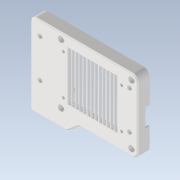
# Autodesk Inventor part: CM4_Case_Buttom
Saved by Autodesk Inventor 2022.1 (Build 261234020, 234B)
## iProperties
Created: 2022-07-26
Part Number: CM4_Case_Buttom
Material: Generisch
Document SubType Name: Modeling
Designer: Rama
Density: 1 g/cm^3
Appearance: Vorgabe
Author: Rama
Autodesk Inventor part; units mm, degrees
ref_plane "YZ Plane" through (0, 0, 0) normal (1, 0, 0) x (0, 1, 0)
ref_plane "XZ Plane" through (0, 0, 0) normal (0, 1, 0) x (-1, 0, 0)
ref_plane "XY Plane" through (0, 0, 0) normal (0, 0, 1) x (1, 0, 0)
sketch "Skizze1" plane through (0, 0, 0) normal (0, 0, 1) x (1, 0, 0)
  circle A0 centre (-59.4355, 41.65) radius 1.35 projected
  circle A1 centre (-59.433, 8.65) radius 1.35 projected
  circle A2 centre (-11.4355, 41.6536) radius 1.35 projected
  circle A3 centre (-11.433, 8.65) radius 1.35 projected
  circle A4 centre (-61.383, 0) radius 1.5 projected
  circle A5 centre (-61.383, 49) radius 1.5 projected
  circle A6 centre (-3.383, 49) radius 1.5 projected
  circle A7 centre (-3.383, 0) radius 1.5 projected
  circle A8 centre (-59.433, 8.65) radius 3.55
  circle A9 centre (-61.383, 0) radius 3.55
  circle A10 centre (-59.4355, 41.65) radius 3.55
  circle A11 centre (-61.383, 49) radius 3.55
  circle A12 centre (-3.383, 49) radius 3.55
  circle A13 centre (-11.4355, 41.6536) radius 3.55
  circle A14 centre (-11.433, 8.65) radius 3.55
  circle A15 centre (-3.383, 0) radius 3.55
  point P0 (0, 0)
  dimension "d0" = 7.1
  dimension "d1" = 7.1
  dimension "d2" = 7.1
  dimension "d3" = 7.1
  dimension "d4" = 7.1
  dimension "d5" = 7.1
  dimension "d6" = 7.1
  dimension "d7" = 7.1
  constraints: 8 centre point, 8 coincident
  measures "d0" diameter of A8
  measures "d1" diameter of A9
  measures "d2" diameter of A10
  measures "d3" diameter of A11
  measures "d4" diameter of A13
  measures "d5" diameter of A12
  measures "d6" diameter of A14
  measures "d7" diameter of A15
extrude "Extrusion1" add sketch "Skizze1" along normal blind 3.8 contours A0 | A1 | A2 | A3 | A4 | A5 | A6 | A7 | A8 | A9 | A10 | A11 | A12 | A13 | A14 | A15
sketch "Skizze2" plane through (-61.383, 0, 3.8) normal (0, 0, 1) x (1, 0, 0)
  line L0 (-20, 52.383) -> (58, 52.3726) projected
  line L1 (-20.5292, 52.3414) -> (-20, 52.383) projected
  line L2 (-21.0454, 52.2175) -> (-20.5292, 52.3414) projected
  line L3 (-21.5359, 52.0143) -> (-21.0454, 52.2175) projected
  line L4 (-21.9885, 51.7369) -> (-21.5359, 52.0143) projected
  line L5 (-22.3922, 51.3922) -> (-21.9885, 51.7369) projected
  line L6 (-22.7369, 50.9885) -> (-22.3922, 51.3922) projected
  line L7 (-23.0143, 50.5359) -> (-22.7369, 50.9885) projected
  line L8 (-23.2175, 50.0454) -> (-23.0143, 50.5359) projected
  line L9 (-23.3414, 49.5292) -> (-23.2175, 50.0454) projected
  line L10 (-23.3726, 49) -> (-23.3414, 49.5292) projected
  line L11 (-23.383, 0) -> (-23.3726, 49) projected
  line L12 (-23.3414, -0.5292) -> (-23.383, 0) projected
  line L13 (-23.2175, -1.0454) -> (-23.3414, -0.5292) projected
  line L14 (-23.0143, -1.5359) -> (-23.2175, -1.0454) projected
  line L15 (-22.7369, -1.9885) -> (-23.0143, -1.5359) projected
  line L16 (-22.3922, -2.3922) -> (-22.7369, -1.9885) projected
  line L17 (-21.9885, -2.7369) -> (-22.3922, -2.3922) projected
  line L18 (-21.5359, -3.0143) -> (-21.9885, -2.7369) projected
  line L19 (-21.0454, -3.2175) -> (-21.5359, -3.0143) projected
  line L20 (-20.5292, -3.3414) -> (-21.0454, -3.2175) projected
  line L21 (-20, -3.3726) -> (-20.5292, -3.3414) projected
  line L22 (58, -3.383) -> (-20, -3.3726) projected
  line L23 (58.5292, -3.3414) -> (58, -3.383) projected
  line L24 (59.0454, -3.2175) -> (58.5292, -3.3414) projected
  line L25 (59.5359, -3.0143) -> (59.0454, -3.2175) projected
  line L26 (59.9885, -2.7369) -> (59.5359, -3.0143) projected
  line L27 (60.3922, -2.3922) -> (59.9885, -2.7369) projected
  line L28 (60.7369, -1.9885) -> (60.3922, -2.3922) projected
  line L29 (61.0143, -1.5359) -> (60.7369, -1.9885) projected
  line L30 (61.2175, -1.0454) -> (61.0143, -1.5359) projected
  line L31 (61.3414, -0.5292) -> (61.2175, -1.0454) projected
  line L32 (61.383, 0) -> (61.3414, -0.5292) projected
  line L33 (61.383, 49) -> (61.3726, 0.0008) projected
  line L34 (61.3414, 49.5292) -> (61.383, 49) projected
  line L35 (61.2175, 50.0454) -> (61.3414, 49.5292) projected
  line L36 (61.0143, 50.5359) -> (61.2175, 50.0454) projected
  line L37 (60.7369, 50.9885) -> (61.0143, 50.5359) projected
  line L38 (60.3922, 51.3922) -> (60.7369, 50.9885) projected
  line L39 (59.9885, 51.7369) -> (60.3922, 51.3922) projected
  line L40 (59.5359, 52.0143) -> (59.9885, 51.7369) projected
  line L41 (59.0454, 52.2175) -> (59.5359, 52.0143) projected
  line L42 (58.5292, 52.3414) -> (59.0454, 52.2175) projected
  line L43 (58, 52.3726) -> (58.5292, 52.3414) projected
  line L44 (-20.3726, -3.683) -> (58.383, -3.683)
  line L45 (61.783, -0.283) -> (61.783, 49.2726)
  line L46 (58.383, 52.6726) -> (-20.3726, 52.6726)
  line L47 (-23.7726, 49.2726) -> (-23.7726, -0.283)
  arc A0 (58.383, -3.683) -> (61.783, -0.283) centre (58.383, -0.283) ccw
  arc A1 (-23.7726, -0.283) -> (-20.3726, -3.683) centre (-20.3726, -0.283) ccw
  arc A2 (-20.3726, 52.6726) -> (-23.7726, 49.2726) centre (-20.3726, 49.2726) ccw
  arc A3 (61.783, 49.2726) -> (58.383, 52.6726) centre (58.383, 49.2726) ccw
  line L48 (-20.3726, -5.283) -> (58.383, -5.283)
  line L49 (63.383, -0.283) -> (63.383, 49.2726)
  line L50 (58.383, 54.2726) -> (-20.3726, 54.2726)
  line L51 (-25.3726, 49.2726) -> (-25.3726, -0.283)
  arc A4 (-25.3726, -0.283) -> (-20.3726, -5.283) centre (-20.3726, -0.283) ccw
  arc A5 (-20.3726, 54.2726) -> (-25.3726, 49.2726) centre (-20.3726, 49.2726) ccw
  arc A6 (63.383, 49.2726) -> (58.383, 54.2726) centre (58.383, 49.2726) ccw
  arc A7 (58.383, -5.283) -> (63.383, -0.283) centre (58.383, -0.283) ccw
  dimension "d11" = 55.7557
  dimension "d12" = 84.7557
  dimension "d13" = 0.4
  dimension "d14" = 0.4
  dimension "d15" = 85.5557
  dimension "d16" = 0.3
  dimension "d17" = 0.3
  dimension "d18" = 56.3557
  dimension "d19" = 3.4
  dimension "d20" = 1.6
  dimension "d21" = 1.6
  dimension "d22" = 1.6
  dimension "d23" = 1.6
  dimension "d25" = 1.6
  constraints: 16 end point, 16 point on circle, 16 tangent, 8 centre point, 6 equal radius, 4 parallel, 2 horizontal, 2 perpendicular
  measures "d11" distance between parallel lines of L22 L0
  measures "d12" distance from line of L10.start L33
  measures "d13" distance from line of L33.start L45
  measures "d14" distance from line of L10.start L47
  measures "d15" distance between parallel lines of L45 L47
  measures "d16" distance from line of L0.end L46
  measures "d17" distance from line of L22.start L44
  measures "d18" distance between parallel lines of L46 L44
  measures "d19" radius of A0
  measures "d20" distance between parallel lines of L47 L51
  measures "d21" distance between parallel lines of L46 L50
  measures "d22" distance between parallel lines of L48 L44
  measures "d23" distance between parallel lines of L45 L49
  measures "d25" radial gap between concentric circles of A4 A1
extrude "Extrusion2" add sketch "Skizze2" against normal blind 5
sketch "Skizze3" plane through (-3.383, 0, 3.8) normal (0, 0, 1) x (1, 0, 0)
  arc A0 (0.383, -5.283) -> (5.383, -0.283) centre (0.383, -0.283) ccw projected
  line L0 (5.383, -0.283) -> (5.383, 49.2726) projected
  arc A1 (5.383, 49.2726) -> (0.383, 54.2726) centre (0.383, 49.2726) ccw projected
  line L1 (0.383, 54.2726) -> (-78.3726, 54.2726) projected
  arc A2 (-78.3726, 54.2726) -> (-83.3726, 49.2726) centre (-78.3726, 49.2726) ccw projected
  line L2 (-83.3726, 49.2726) -> (-83.3726, -0.283) projected
  arc A3 (-83.3726, -0.283) -> (-78.3726, -5.283) centre (-78.3726, -0.283) ccw projected
  line L3 (-78.3726, -5.283) -> (0.383, -5.283) projected
  arc A4 (-81.7726, -0.283) -> (-78.3726, -3.683) centre (-78.3726, -0.283) ccw projected
  line L4 (-81.7726, -0.283) -> (-81.7726, 49.2726) projected
  arc A5 (-78.3726, 52.6726) -> (-81.7726, 49.2726) centre (-78.3726, 49.2726) ccw projected
  line L5 (-78.3726, 52.6726) -> (0.383, 52.6726) projected
  arc A6 (3.783, 49.2726) -> (0.383, 52.6726) centre (0.383, 49.2726) ccw projected
  line L6 (3.783, 49.2726) -> (3.783, -0.283) projected
  arc A7 (0.383, -3.683) -> (3.783, -0.283) centre (0.383, -0.283) ccw projected
  line L7 (0.383, -3.683) -> (-78.3726, -3.683) projected
  line L8 (-52.2525, 5.75) -> (-11.8525, 5.75)
  line L9 (-11.8525, 5.75) -> (-11.8525, 46.15)
  line L10 (-11.8525, 46.15) -> (-52.2525, 46.15)
  line L11 (-52.2525, 46.15) -> (-52.2525, 5.75)
  circle A8 centre (-15.62, 25.95) radius 2.1 projected
  line L12 (-50.2525, 5.75) -> (-49.0525, 5.75)
  line L13 (-49.0525, 5.75) -> (-49.0525, 46.15)
  line L14 (-49.0525, 46.15) -> (-50.2525, 46.15)
  line L15 (-50.2525, 46.15) -> (-50.2525, 5.75)
  line L16 (-47.0525, 46.15) -> (-45.8525, 46.15)
  line L17 (-45.8525, 46.15) -> (-45.8525, 5.75)
  line L18 (-45.8525, 5.75) -> (-47.0525, 5.75)
  line L19 (-47.0525, 5.75) -> (-47.0525, 46.15)
  line L20 (-43.8525, 5.75) -> (-42.6525, 5.75)
  line L21 (-42.6525, 5.75) -> (-42.6525, 46.15)
  line L22 (-42.6525, 46.15) -> (-43.8525, 46.15)
  line L23 (-43.8525, 46.15) -> (-43.8525, 5.75)
  line L24 (-40.6525, 46.15) -> (-39.4525, 46.15)
  line L25 (-39.4525, 46.15) -> (-39.4525, 5.75)
  line L26 (-39.4525, 5.75) -> (-40.6525, 5.75)
  line L27 (-40.6525, 5.75) -> (-40.6525, 46.15)
  line L28 (-37.4525, 5.75) -> (-36.2525, 5.75)
  line L29 (-36.2525, 5.75) -> (-36.2525, 46.15)
  line L30 (-36.2525, 46.15) -> (-37.4525, 46.15)
  line L31 (-37.4525, 46.15) -> (-37.4525, 5.75)
  line L32 (-34.2525, 46.15) -> (-33.0525, 46.15)
  line L33 (-33.0525, 46.15) -> (-33.0525, 5.75)
  line L34 (-33.0525, 5.75) -> (-34.2525, 5.75)
  line L35 (-34.2525, 5.75) -> (-34.2525, 46.15)
  line L36 (-31.0525, 5.75) -> (-29.8525, 5.75)
  line L37 (-29.8525, 5.75) -> (-29.8525, 46.15)
  line L38 (-29.8525, 46.15) -> (-31.0525, 46.15)
  line L39 (-31.0525, 46.15) -> (-31.0525, 5.75)
  line L40 (-27.8525, 46.15) -> (-26.6525, 46.15)
  line L41 (-26.6525, 46.15) -> (-26.6525, 5.75)
  line L42 (-26.6525, 5.75) -> (-27.8525, 5.75)
  line L43 (-27.8525, 5.75) -> (-27.8525, 46.15)
  line L44 (-24.6525, 5.75) -> (-23.4525, 5.75)
  line L45 (-23.4525, 5.75) -> (-23.4525, 46.15)
  line L46 (-23.4525, 46.15) -> (-24.6525, 46.15)
  line L47 (-24.6525, 46.15) -> (-24.6525, 5.75)
  line L48 (-21.4525, 46.15) -> (-20.2525, 46.15)
  line L49 (-20.2525, 46.15) -> (-20.2525, 5.75)
  line L50 (-20.2525, 5.75) -> (-21.4525, 5.75)
  line L51 (-21.4525, 5.75) -> (-21.4525, 46.15)
  line L52 (-18.2525, 5.75) -> (-17.0525, 5.75)
  line L53 (-17.0525, 5.75) -> (-17.0525, 46.15)
  line L54 (-17.0525, 46.15) -> (-18.2525, 46.15)
  line L55 (-18.2525, 46.15) -> (-18.2525, 5.75)
  line L56 (-15.0525, 5.75) -> (-13.8525, 5.75)
  line L57 (-13.8525, 5.75) -> (-13.8525, 46.15)
  line L58 (-13.8525, 46.15) -> (-15.0525, 46.15)
  line L59 (-15.0525, 46.15) -> (-15.0525, 5.75)
  circle A9 centre (-56.0525, 41.65) radius 3.55 projected
  circle A10 centre (-8.0525, 41.6536) radius 3.55 projected
  point P0 (3.383, 0)
  point P1 (-52.2525, 25.95)
  point P2 (-32.0525, 5.75)
  point P3 (-11.8525, 25.95)
  point P4 (-33.6525, 46.15)
  point P5 (-30.4525, 46.15)
  point P6 (-27.2525, 46.15)
  point P7 (-24.0525, 46.15)
  point P8 (-20.8525, 46.15)
  point P9 (-17.6525, 46.15)
  point P10 (-36.8525, 46.15)
  point P11 (-40.0525, 46.15)
  point P12 (-43.2525, 46.15)
  point P13 (-46.4525, 46.15)
  point P14 (-49.6525, 46.15)
  point P15 (-14.4525, 46.15)
  dimension "d28" = 40.4
  dimension "d29" = 40.4
  dimension "d38" = 0
  dimension "d39" = 1.2
  dimension "d40" = 1.2
  dimension "d41" = 1.2
  dimension "d42" = 1.2
  dimension "d43" = 1.2
  dimension "d44" = 1.2
  dimension "d45" = 1.2
  dimension "d46" = 1.2
  dimension "d47" = 1.2
  dimension "d48" = 1.2
  dimension "d49" = 1.2
  dimension "d54" = 3.2
  dimension "d55" = 3.2
  dimension "d56" = 3.2
  dimension "d57" = 3.2
  dimension "d58" = 3.2
  dimension "d59" = 3.2
  dimension "d60" = 3.2
  dimension "d61" = 3.2
  dimension "d62" = 3.2
  dimension "d63" = 3.2
  dimension "d64" = 1.2
  dimension "d65" = 3.2
  dimension "d66" = 2
  dimension "d67" = 2
  dimension "d69" = 3.8
  dimension "d70" = 3.8
  constraints: 100 end point, 25 parallel, 14 midpoint, 12 horizontal, 12 perpendicular, 1 vertical, 31 other
  measures "d28" distance of L11.start L9.end
  measures "d29" distance of L9.end L9.start
  measures "d38" vertical distance of A8.centre point (-11.852, 25.95)
  measures "d39" distance between parallel lines of L13 L15
  measures "d40" distance between parallel lines of L17 L19
  measures "d41" distance between parallel lines of L21 L23
  measures "d42" distance between parallel lines of L25 L27
  measures "d43" distance between parallel lines of L29 L31
  measures "d44" distance between parallel lines of L33 L35
  measures "d45" distance between parallel lines of L37 L39
  measures "d46" distance between parallel lines of L41 L43
  measures "d47" distance between parallel lines of L45 L47
  measures "d48" distance between parallel lines of L49 L51
  measures "d49" distance between parallel lines of L53 L55
  measures "d54" distance of point (-33.652, 46.15) point (-30.452, 46.15)
  measures "d55" distance of point (-30.452, 46.15) point (-27.252, 46.15)
  measures "d56" distance of point (-27.252, 46.15) point (-24.052, 46.15)
  measures "d57" distance of point (-24.052, 46.15) point (-20.852, 46.15)
  measures "d58" distance of point (-20.852, 46.15) point (-17.652, 46.15)
  measures "d59" distance of point (-36.852, 46.15) point (-33.652, 46.15)
  measures "d60" distance of point (-40.052, 46.15) point (-36.852, 46.15)
  measures "d61" distance of point (-43.252, 46.15) point (-40.052, 46.15)
  measures "d62" distance of point (-46.452, 46.15) point (-43.252, 46.15)
  measures "d63" distance of point (-49.652, 46.15) point (-46.452, 46.15)
  measures "d64" distance between parallel lines of L57 L59
  measures "d65" distance of point (-17.652, 46.15) point (-14.452, 46.15)
  measures "d66" distance between parallel lines of L11 L15
  measures "d67" distance between parallel lines of L57 L9
  measures "d69" distance from line of A10.centre L9
  measures "d70" distance from line of A9.centre L11
extrude "Extrusion3" add sketch "Skizze3" along normal blind 2.6 contours L3 A3 L2 A2 L1 A1 L0 A0 | L4 A5 L5 A6 L6 A7 L7 A4 | A9 | A10
sketch "Skizze4" plane through (-3.383, 0, 6.4) normal (0, 0, 1) x (1, 0, 0)
  line L0 (-49.0525, 5.75) -> (-49.0525, 46.15) projected
  line L1 (-50.2525, 46.15) -> (-50.2525, 5.75) projected
  line L2 (5.383, -0.283) -> (5.383, 49.2726) projected
  arc A0 (5.383, 49.2726) -> (0.383, 54.2726) centre (0.383, 49.2726) ccw projected
  line L3 (0.383, 54.2726) -> (-78.3726, 54.2726) projected
  arc A1 (-78.3726, 54.2726) -> (-83.3726, 49.2726) centre (-78.3726, 49.2726) ccw projected
  line L4 (-83.3726, 49.2726) -> (-83.3726, -0.283) projected
  arc A2 (-83.3726, -0.283) -> (-78.3726, -5.283) centre (-78.3726, -0.283) ccw projected
  line L5 (-78.3726, -5.283) -> (0.383, -5.283) projected
  arc A3 (0.383, -5.283) -> (5.383, -0.283) centre (0.383, -0.283) ccw projected
  line L6 (-11.8525, 46.15) -> (-11.8525, 5.75) projected
  line L7 (-11.8525, 5.75) -> (-52.2525, 5.75) projected
  line L8 (-52.2525, 5.75) -> (-52.2525, 46.15) projected
  line L9 (-52.2525, 46.15) -> (-11.8525, 46.15) projected
  line L10 (-47.0525, 5.75) -> (-47.0525, 46.15) projected
  line L11 (-45.8525, 46.15) -> (-45.8525, 5.75) projected
  line L12 (-43.8525, 46.15) -> (-43.8525, 5.75) projected
  line L13 (-42.6525, 5.75) -> (-42.6525, 46.15) projected
  line L14 (-40.6525, 5.75) -> (-40.6525, 46.15) projected
  line L15 (-39.4525, 46.15) -> (-39.4525, 5.75) projected
  line L16 (-37.4525, 46.15) -> (-37.4525, 5.75) projected
  line L17 (-36.2525, 5.75) -> (-36.2525, 46.15) projected
  line L18 (-34.2525, 5.75) -> (-34.2525, 46.15) projected
  line L19 (-33.0525, 46.15) -> (-33.0525, 5.75) projected
  line L20 (-31.0525, 46.15) -> (-31.0525, 5.75) projected
  line L21 (-29.8525, 5.75) -> (-29.8525, 46.15) projected
  line L22 (-27.8525, 5.75) -> (-27.8525, 46.15) projected
  line L23 (-26.6525, 46.15) -> (-26.6525, 5.75) projected
  line L24 (-24.6525, 46.15) -> (-24.6525, 5.75) projected
  line L25 (-23.4525, 5.75) -> (-23.4525, 46.15) projected
  line L26 (-21.4525, 5.75) -> (-21.4525, 46.15) projected
  line L27 (-20.2525, 46.15) -> (-20.2525, 5.75) projected
  line L28 (-18.2525, 46.15) -> (-18.2525, 5.75) projected
  line L29 (-17.0525, 5.75) -> (-17.0525, 46.15) projected
  line L30 (-15.0525, 46.15) -> (-15.0525, 5.75) projected
  line L31 (-13.8525, 5.75) -> (-13.8525, 46.15) projected
  point P0 (3.383, 0)
  point P1 (-49.0525, 5.75)
  point P2 (-50.2525, 5.75)
  constraints: 2 other
extrude "Extrusion4" add sketch "Skizze4" along normal blind 2.2 contours L7 L1 L9 L0 | L10 L9 L11 L7 | L12 L9 L13 L7 | L14 L9 L15 L7 | L16 L9 L17 L7 | L18 L9 L19 L7 | L20 L9 L21 L7 | L22 L9 L23 L7 | L24 L9 L25 L7 | L26 L9 L27 L7 | L28 L9 L29 L7 | L30 L9 L31 L7 | A3 L5 A2 L4 A1 L3 A0 L2
sketch "Skizze5" plane through (-3.383, 0, 8.6) normal (0, 0, 1) x (1, 0, 0)
  circle A0 centre (0, 0) radius 3.55 projected
  circle A1 centre (-58, 0) radius 3.55 projected
  circle A2 centre (-56.05, 8.65) radius 3.55 projected
  circle A3 centre (0, 49) radius 3.55 projected
  circle A4 centre (-8.0525, 41.6536) radius 3.55 projected
  circle A5 centre (-56.0525, 41.65) radius 3.55 projected
  circle A6 centre (-58, 49) radius 3.55 projected
  circle A7 centre (-8.05, 8.65) radius 3.55 projected
  point P0 (3.383, 0)
hole "Bohrung1" at (-61.383, 0, 8.6) at (-3.383, 0, 8.6) at (-3.383, 49, 8.6) at (-61.383, 49, 8.6) direction (0, 0, -1) diameter 3.3 end through all counterbore diameter 4.7 counterbore depth 5
hole "Bohrung2" at (-59.4355, 41.65, 8.6) at (-59.433, 8.65, 8.6) at (-11.433, 8.65, 8.6) at (-11.4355, 41.6536, 8.6) direction (0, 0, -1) diameter 2.5 end through all
sketch "Skizze6" plane through (-3.383, 0, 3.8) normal (0, 0, -1) x (-1, 0, 0)
  line L0 (75.3726, 42.6448) -> (1.617, 42.6448)
  line L1 (1.617, 42.6448) -> (1.617, 11.1448)
  line L2 (1.617, 11.1448) -> (75.3726, 11.1448)
  line L3 (75.3726, 11.1448) -> (75.3726, 42.6448)
  line L4 (-5.383, 49.2726) -> (-5.383, -0.283) projected
  line L5 (83.3726, -0.283) -> (83.3726, 49.2726) projected
  point P0 (-3.383, 0)
  point P1 (-5.383, 24.4948)
  point P2 (1.617, 26.8948)
  point P3 (-5.383, 24.4948)
  dimension "d89" = 31.5
  dimension "d91" = 7
  dimension "d92" = 8
  dimension "d93" = 2.4
  constraints: 8 end point, 3 midpoint, 2 parallel, 1 horizontal, 1 perpendicular
  measures "d89" distance of L1.end L0.end
  measures "d91" distance between parallel lines of L4 L1
  measures "d92" distance between parallel lines of L5 L3
  measures "d93" vertical distance of point (1.617, 26.895) point (-5.383, 24.495)
hole "Bohrung3" at (-5, 42.6448, 3.8) at (-5, 11.1448, 3.8) at (-78.7557, 11.1448, 3.8) at (-78.7557, 42.6448, 3.8) direction (0, 0, 1) diameter 3.3 end through all counterbore diameter 5.8 counterbore depth 3.2
chamfer "Fase1" distance 0.4 angle 45 36 edges at (-62.983, 8.65, 0) (-64.933, 0, 0) (-62.9855, 41.65, 0) (-64.933, 49, 0) (-14.9855, 41.6536, 0) (-6.933, 49, 0) (-14.983, 8.65, 0) (-6.933, 0, 0) (-18.4355, 25.95, 6.4) (-17.2355, 25.95, 6.4) (-21.6355, 25.95, 6.4) (-20.4355, 25.95, 6.4) (-15.2355, 25.95, 3.8) (-35.4355, 46.15, 3.8) (-35.4355, 5.75, 3.8) (-55.6355, 25.95, 3.8) (-23.6355, 25.95, 6.4) (-24.8355, 25.95, 6.4) (-28.0355, 25.95, 6.4) (-26.8355, 25.95, 6.4) (-31.2355, 25.95, 6.4) (-30.0355, 25.95, 6.4) (-34.4355, 25.95, 6.4) (-33.2355, 25.95, 6.4) (-37.6355, 25.95, 6.4) (-36.4355, 25.95, 6.4) (-40.8355, 25.95, 6.4) (-39.6355, 25.95, 6.4) (-44.0355, 25.95, 6.4) (-42.8355, 25.95, 6.4) (-47.2355, 25.95, 6.4) (-46.0355, 25.95, 6.4) (-50.4355, 25.95, 6.4) (-49.2355, 25.95, 6.4) (-52.4355, 25.95, 6.4) (-53.6355, 25.95, 6.4)
chamfer "Fase2" distance 0.4 angle 45 52 edges at (-53.6355, 25.95, 8.6) (-52.4355, 25.95, 8.6) (-50.4355, 25.95, 8.6) (-49.2355, 25.95, 8.6) (-47.2355, 25.95, 8.6) (-46.0355, 25.95, 8.6) (-44.0355, 25.95, 8.6) (-42.8355, 25.95, 8.6) (-40.8355, 25.95, 8.6) (-39.6355, 25.95, 8.6) (-37.6355, 25.95, 8.6) (-36.4355, 25.95, 8.6) (-34.4355, 25.95, 8.6) (-33.2355, 25.95, 8.6) (-31.2355, 25.95, 8.6) (-30.0355, 25.95, 8.6) (-28.0355, 25.95, 8.6) (-26.8355, 25.95, 8.6) (-24.8355, 25.95, 8.6) (-23.6355, 25.95, 8.6) (-21.6355, 25.95, 8.6) (-20.4355, 25.95, 8.6) (-18.4355, 25.95, 8.6) (-17.2355, 25.95, 8.6) (-15.2355, 25.95, 8.6) (-55.6355, 25.95, 8.6) (-54.6355, 5.75, 8.6) (-51.4355, 5.75, 8.6) (-48.2355, 5.75, 8.6) (-45.0355, 5.75, 8.6) (-41.8355, 5.75, 8.6) (-38.6355, 5.75, 8.6) (-35.4355, 5.75, 8.6) (-32.2355, 5.75, 8.6) (-29.0355, 5.75, 8.6) (-25.8355, 5.75, 8.6) (-22.6355, 5.75, 8.6) (-19.4355, 5.75, 8.6) (-16.2355, 5.75, 8.6) (-16.2355, 46.15, 8.6) (-19.4355, 46.15, 8.6) (-22.6355, 46.15, 8.6) (-25.8355, 46.15, 8.6) (-29.0355, 46.15, 8.6) (-32.2355, 46.15, 8.6) (-35.4355, 46.15, 8.6) (-38.6355, 46.15, 8.6) (-41.8355, 46.15, 8.6) (-45.0355, 46.15, 8.6) (-48.2355, 46.15, 8.6) (-51.4355, 46.15, 8.6) (-54.6355, 46.15, 8.6)
sketch "Skizze7" plane through (-61.383, 0, -1.2) normal (0, 0, -1) x (-1, 0, 0)
  arc A0 (-63.383, -0.283) -> (-58.383, -5.283) centre (-58.383, -0.283) ccw projected
  line L0 (-58.383, -5.283) -> (20.3726, -5.283) projected
  arc A1 (20.3726, -5.283) -> (25.3726, -0.283) centre (20.3726, -0.283) ccw projected
  line L1 (25.3726, -0.283) -> (25.3726, 49.2726) projected
  arc A2 (25.3726, 49.2726) -> (20.3726, 54.2726) centre (20.3726, 49.2726) ccw projected
  line L2 (20.3726, 54.2726) -> (-58.383, 54.2726) projected
  arc A3 (-58.383, 54.2726) -> (-63.383, 49.2726) centre (-58.383, 49.2726) ccw projected
  line L3 (-63.383, 49.2726) -> (-63.383, -0.283) projected
  arc A4 (20.3726, -3.683) -> (23.7726, -0.283) centre (20.3726, -0.283) ccw projected
  line L4 (20.3726, -3.683) -> (-58.383, -3.683) projected
  arc A5 (-61.783, -0.283) -> (-58.383, -3.683) centre (-58.383, -0.283) ccw projected
  line L5 (-61.783, -0.283) -> (-61.783, 49.2726) projected
  arc A6 (-58.383, 52.6726) -> (-61.783, 49.2726) centre (-58.383, 49.2726) ccw projected
  line L6 (-58.383, 52.6726) -> (20.3726, 52.6726) projected
  arc A7 (23.7726, 49.2726) -> (20.3726, 52.6726) centre (20.3726, 49.2726) ccw projected
  line L7 (23.7726, 49.2726) -> (23.7726, -0.283) projected
  line L8 (25.3726, 49.2726) -> (25.3726, -0.283) projected
  line L9 (25.3726, 6.4318) -> (-5.8274, 6.4318)
  line L10 (-5.8274, 6.4318) -> (-5.8274, -13.283)
  line L11 (-5.8274, -13.283) -> (25.3726, -13.283)
  line L12 (25.3726, -13.283) -> (25.3726, 6.4318)
  line L13 (23.7726, 49.2726) -> (23.7726, -0.283) projected
  line L14 (23.7726, 8.4987) -> (-4.2274, 8.4987)
  line L15 (-4.2274, 8.4987) -> (-4.2274, -11.683)
  line L16 (-4.2274, -11.683) -> (23.7726, -11.683)
  line L17 (23.7726, -11.683) -> (23.7726, 8.4987)
  line L18 (23.7726, -9.883) -> (-4.2274, -9.883)
  point P0 (-61.383, 0)
  point P1 (-5.8274, -5.283)
  point P2 (25.3726, -0.283)
  dimension "d107" = 8
  dimension "d108" = 29.6
  dimension "d109" = 1.6
  dimension "d110" = 1.6
  dimension "d111" = 1.8
  dimension "d114" = 1.6
  constraints: 18 end point, 4 parallel, 4 point on line, 3 perpendicular, 2 horizontal
  measures "d107" distance between parallel lines of L0 L11
  measures "d108" distance between parallel lines of L7 L10
  measures "d109" distance between parallel lines of L10 L15
  measures "d110" distance between parallel lines of L11 L16
  measures "d111" distance between parallel lines of L16 L18
  measures "d114" distance between parallel lines of L4 L0
extrude "Extrusion5" add sketch "Skizze7" against normal blind 3.2 contours L0 L15 L16 L17 A1 L12 L11 L10 | L0 A1 L17 L18 L15
sketch "Skizze8" plane through (-61.383, 0, -1.2) normal (0, 0, -1) x (-1, 0, 0)
  line L0 (23.7726, -9.883) -> (-4.2274, -9.883) projected
  line L1 (6.3726, -9.883) -> (0.5726, -9.883)
  line L2 (0.5726, -9.883) -> (0.5726, -7.283)
  line L3 (0.5726, -7.283) -> (6.3726, -7.283)
  line L4 (6.3726, -7.283) -> (6.3726, -9.883)
  line L5 (23.7726, -9.883) -> (23.7726, -11.683) projected
  line L6 (-4.2274, -11.683) -> (-4.2274, -9.883) projected
  line L7 (23.7726, -11.683) -> (-4.2274, -11.683) projected
  point P0 (-61.383, 0)
  point P1 (0.5726, -9.883)
  dimension "d115" = 17.4
  dimension "d116" = 4.8
  dimension "d117" = 4.4
  constraints: 8 end point, 2 parallel, 1 horizontal, 1 perpendicular, 1 point on line
  measures "d115" distance between parallel lines of L5 L4
  measures "d116" distance between parallel lines of L6 L2
  measures "d117" distance between parallel lines of L7 L3
extrude "Extrusion6" cut sketch "Skizze8" against normal through all contours L0 L2 L3 L4
sketch "Skizze9" plane through (-61.383, 0, 2) normal (0, 0, 1) x (1, 0, 0)
  line L0 (-6.3726, -9.883) -> (-6.3726, -7.283) projected
  line L1 (-6.3726, -7.283) -> (-0.5726, -7.283) projected
  line L2 (-0.5726, -7.283) -> (-0.5726, -9.883) projected
  line L3 (-0.5726, -9.883) -> (4.2274, -9.883) projected
  line L4 (4.2274, -9.883) -> (4.2274, -11.683) projected
  line L5 (4.2274, -11.683) -> (-23.7726, -11.683) projected
  line L6 (-23.7726, -11.683) -> (-23.7726, -9.883) projected
  line L7 (-23.7726, -9.883) -> (-6.3726, -9.883) projected
  line L8 (5.8274, -13.283) -> (5.8274, -5.283) projected
  line L9 (-20.3726, -5.283) -> (5.8274, -5.283) projected
  arc A0 (-25.3726, -0.283) -> (-20.3726, -5.283) centre (-20.3726, -0.283) ccw projected
  line L10 (-25.3726, -0.283) -> (-25.3726, -13.283) projected
  line L11 (-25.3726, -13.283) -> (5.8274, -13.283) projected
  point P0 (61.383, 0)
extrude "Extrusion7" add sketch "Skizze9" along normal up to surface (6.6 mm away) contours L0 L1 L2 L3 L4 L5 L6 L7 | L11 L10 A0 L9 L8
fillet "Rundung1" radius 3 1 edges at (-55.5557, -5.283, 3.7)
fillet "Rundung2" radius 1.6 2 edges at (-55.5557, -13.283, 3.7) (-86.7557, -13.283, 3.7)
sketch "Skizze10" plane through (-3.383, 0, 8.6) normal (0, 0, 1) x (1, 0, 0)
  arc A0 (-83.3726, -11.683) -> (-81.7726, -13.283) centre (-81.7726, -11.683) ccw projected
  line L0 (-53.7726, -13.283) -> (-81.7726, -13.283) projected
  arc A1 (-53.7726, -13.283) -> (-52.1726, -11.683) centre (-53.7726, -11.683) ccw projected
  line L1 (-52.1726, -8.283) -> (-52.1726, -11.683) projected
  arc A2 (-49.1726, -5.283) -> (-52.1726, -8.283) centre (-49.1726, -8.283) ccw projected
  line L2 (-49.1726, -5.283) -> (0.383, -5.283) projected
  arc A3 (0.383, -5.283) -> (5.383, -0.283) centre (0.383, -0.283) ccw projected
  line L3 (5.383, -0.283) -> (5.383, 49.2726) projected
  arc A4 (5.383, 49.2726) -> (0.383, 54.2726) centre (0.383, 49.2726) ccw projected
  line L4 (0.383, 54.2726) -> (-78.3726, 54.2726) projected
  arc A5 (-78.3726, 54.2726) -> (-83.3726, 49.2726) centre (-78.3726, 49.2726) ccw projected
  line L5 (-83.3726, 49.2726) -> (-83.3726, -11.683) projected
  line L6 (-11.4525, 5.35) -> (-11.4525, 46.55) projected
  line L7 (-14.2525, 5.35) -> (-11.4525, 5.35) projected
  line L8 (-14.2525, 46.55) -> (-14.2525, 5.35) projected
  line L9 (-11.4525, 46.55) -> (-14.2525, 46.55) projected
  line L10 (-17.8525, 5.35) -> (-17.8525, 46.55) projected
  line L11 (-20.6525, 5.35) -> (-17.8525, 5.35) projected
  line L12 (-20.6525, 46.55) -> (-20.6525, 5.35) projected
  line L13 (-17.8525, 46.55) -> (-20.6525, 46.55) projected
  line L14 (-24.2525, 5.35) -> (-24.2525, 46.55) projected
  line L15 (-27.0525, 5.35) -> (-24.2525, 5.35) projected
  line L16 (-27.0525, 46.55) -> (-27.0525, 5.35) projected
  line L17 (-24.2525, 46.55) -> (-27.0525, 46.55) projected
  line L18 (-30.6525, 5.35) -> (-30.6525, 46.55) projected
  line L19 (-33.4525, 5.35) -> (-30.6525, 5.35) projected
  line L20 (-33.4525, 46.55) -> (-33.4525, 5.35) projected
  line L21 (-30.6525, 46.55) -> (-33.4525, 46.55) projected
  line L22 (-37.0525, 5.35) -> (-37.0525, 46.55) projected
  line L23 (-39.8525, 5.35) -> (-37.0525, 5.35) projected
  line L24 (-39.8525, 46.55) -> (-39.8525, 5.35) projected
  line L25 (-37.0525, 46.55) -> (-39.8525, 46.55) projected
  line L26 (-43.4525, 5.35) -> (-43.4525, 46.55) projected
  line L27 (-46.2525, 5.35) -> (-43.4525, 5.35) projected
  line L28 (-46.2525, 46.55) -> (-46.2525, 5.35) projected
  line L29 (-43.4525, 46.55) -> (-46.2525, 46.55) projected
  line L30 (-52.6525, 46.55) -> (-52.6525, 5.35) projected
  line L31 (-49.8525, 46.55) -> (-52.6525, 46.55) projected
  line L32 (-49.8525, 5.35) -> (-49.8525, 46.55) projected
  line L33 (-52.6525, 5.35) -> (-49.8525, 5.35) projected
  circle A6 centre (-75.3726, 11.1448) radius 1.65 projected
  circle A7 centre (-1.617, 42.6448) radius 1.65 projected
  circle A8 centre (-1.617, 11.1448) radius 1.65 projected
  circle A9 centre (-75.3726, 42.6448) radius 1.65 projected
  circle A10 centre (-8.05, 8.65) radius 1.25 projected
  circle A11 centre (-56.0525, 41.65) radius 1.25 projected
  circle A12 centre (-56.05, 8.65) radius 1.25 projected
  circle A13 centre (-8.0525, 41.6536) radius 1.25 projected
  circle A14 centre (0, 49) radius 2.35 projected
  circle A15 centre (-58, 0) radius 2.35 projected
  circle A16 centre (0, 0) radius 2.35 projected
  circle A17 centre (-58, 49) radius 2.35 projected
  line L34 (-46.6525, 5.35) -> (-46.6525, 46.55) projected
  line L35 (-49.4525, 5.35) -> (-46.6525, 5.35) projected
  line L36 (-49.4525, 46.55) -> (-49.4525, 5.35) projected
  line L37 (-46.6525, 46.55) -> (-49.4525, 46.55) projected
  line L38 (-40.2525, 5.35) -> (-40.2525, 46.55) projected
  line L39 (-43.0525, 5.35) -> (-40.2525, 5.35) projected
  line L40 (-43.0525, 46.55) -> (-43.0525, 5.35) projected
  line L41 (-40.2525, 46.55) -> (-43.0525, 46.55) projected
  line L42 (-33.8525, 5.35) -> (-33.8525, 46.55) projected
  line L43 (-36.6525, 5.35) -> (-33.8525, 5.35) projected
  line L44 (-36.6525, 46.55) -> (-36.6525, 5.35) projected
  line L45 (-33.8525, 46.55) -> (-36.6525, 46.55) projected
  line L46 (-27.4525, 5.35) -> (-27.4525, 46.55) projected
  line L47 (-30.2525, 5.35) -> (-27.4525, 5.35) projected
  line L48 (-30.2525, 46.55) -> (-30.2525, 5.35) projected
  line L49 (-27.4525, 46.55) -> (-30.2525, 46.55) projected
  line L50 (-21.0525, 5.35) -> (-21.0525, 46.55) projected
  line L51 (-23.8525, 5.35) -> (-21.0525, 5.35) projected
  line L52 (-23.8525, 46.55) -> (-23.8525, 5.35) projected
  line L53 (-21.0525, 46.55) -> (-23.8525, 46.55) projected
  line L54 (-14.6525, 5.35) -> (-14.6525, 46.55) projected
  line L55 (-17.4525, 5.35) -> (-14.6525, 5.35) projected
  line L56 (-17.4525, 46.55) -> (-17.4525, 5.35) projected
  line L57 (-14.6525, 46.55) -> (-17.4525, 46.55) projected
  line L58 (0.9112, 45.9847) -> (5.383, 45.9847) projected
  line L59 (5.383, 49.2726) -> (5.383, 45.9847) projected
  arc A18 (5.383, 49.2726) -> (0.383, 54.2726) centre (0.383, 49.2726) ccw projected
  line L60 (-3.0834, 54.2726) -> (0.383, 54.2726) projected
  line L61 (-3.0834, 54.2726) -> (-3.0834, 49.6442) projected
  arc A19 (0.9112, 45.9847) -> (-3.0834, 49.6442) centre (0, 49) ccw projected
  line L62 (-41.7726, -3.683) -> (-3.15, -3.683) projected
  arc A20 (-41.7726, -3.683) -> (-44.6679, -4.7085) centre (-41.7726, -8.283) ccw projected
  line L63 (-53.3873, -11.771) -> (-44.6679, -4.7085) projected
  arc A21 (-54.2685, -12.083) -> (-53.3873, -11.771) centre (-54.2685, -10.683) ccw projected
  line L64 (-81.7726, -12.083) -> (-54.2685, -12.083) projected
  line L65 (-81.7726, -9.883) -> (-81.7726, -12.083) projected
  line L66 (-81.7726, -9.883) -> (-83.3726, -9.883) projected
  line L67 (-83.3726, -12.083) -> (-83.3726, -9.883) projected
  arc A22 (-83.3726, -12.083) -> (-81.7726, -13.683) centre (-81.7726, -12.083) ccw projected
  line L68 (-54.2685, -13.683) -> (-81.7726, -13.683) projected
  arc A23 (-54.2685, -13.683) -> (-52.3803, -13.0143) centre (-54.2685, -10.683) ccw projected
  line L69 (-43.6608, -5.9518) -> (-52.3803, -13.0143) projected
  arc A24 (-41.7726, -5.283) -> (-43.6608, -5.9518) centre (-41.7726, -8.283) ccw projected
  line L70 (0.383, -5.283) -> (-41.7726, -5.283) projected
  arc A25 (0.383, -5.283) -> (5.383, -0.283) centre (0.383, -0.283) ccw projected
  line L71 (5.383, 36.6777) -> (5.383, -0.283) projected
  line L72 (3.783, 36.6777) -> (5.383, 36.6777) projected
  line L73 (3.783, 3.15) -> (3.783, 36.6777) projected
  line L74 (3.783, 3.15) -> (0, 3.15) projected
  arc A26 (-3.15, 0) -> (0, 3.15) centre (0, 0) ccw projected
  line L75 (-3.15, 0) -> (-3.15, -3.683) projected
  point P0 (3.383, 0)
  point P1 (-45.3772, -5.283)
  point P2 (-52.1726, -10.7871)
extrude "Extrusion8" add sketch "Skizze10" against normal up to surface (9.8 mm away) contours A0 L0 A1 L1 L63 L2 A24 L69 A23 L68 A22 L67
sketch "Skizze12" plane through (-3.383, 0, 3.8) normal (0, 0, -1) x (-1, 0, 0)
  arc A0 (52.1726, -8.283) -> (49.1726, -5.283) centre (49.1726, -8.283) ccw projected
  line L0 (49.1726, -5.283) -> (-0.383, -5.283) projected
  line L1 (53.2788, -11.683) -> (53.3873, -11.771) projected
  line L2 (52.1726, -8.283) -> (52.1726, -10.7871) projected
  arc A1 (52.1726, -8.283) -> (49.1726, -5.283) centre (49.1726, -8.283) ccw projected
  line L3 (45.3772, -5.283) -> (49.1726, -5.283) projected
  line L4 (44.6679, -4.7085) -> (52.9726, -11.4351) projected
  point P0 (-3.383, 0)
  point P1 (52.1726, -3.683)
  point P2 (52.1726, -11.683)
extrude "Extrusion10" add sketch "Skizze12" against normal up to surface (4.8 mm away)
move faces "Verschieben1" translate (0, 0, 1) faces at (-70.0223, -11.083, 2)
chamfer "Fase4" distance 1 angle 45 7 edges at (-42.3778, 54.2726, 8.6) (-85.2912, 52.8082, 8.6) (-86.7557, 18.5948, 8.6) (-24.0778, -5.283, 8.6) (0.5355, -3.8186, 8.6) (2, 24.4948, 8.6) (0.5355, 52.8082, 8.6)
chamfer "Fase5" distance 0.6 angle 45 4 edges at (-59.4355, 42.9, 0) (-59.433, 9.9, 0) (-11.433, 9.9, 0) (-11.4355, 42.9036, 0)
sketch "Skizze13" plane through (-61.383, 0, -1.2) normal (0, 0, -1) x (-1, 0, 0)
  line L0 (-60.7952, 14.6356) -> (-48.019, 14.6356) projected
  line L1 (-60.7952, 21.8746) -> (-60.7952, 14.6356) projected
  line L2 (-61.8366, 22.916) -> (-60.7952, 21.8746) projected
  line L3 (-61.8366, 29.0882) -> (-61.8366, 22.916) projected
  line L4 (-48.019, 29.0882) -> (-61.8366, 29.0882) projected
  line L5 (-48.019, 14.6356) -> (-48.019, 29.0882) projected
  line L6 (-5.8274, -8.283) -> (-5.8274, -10.7871) projected
  line L7 (20.3726, -3.683) -> (-58.383, -3.683) projected
  arc A0 (-61.783, -0.283) -> (-58.383, -3.683) centre (-58.383, -0.283) ccw projected
  line L8 (-61.783, -0.283) -> (-61.783, 49.2726) projected
  arc A1 (-58.383, 52.6726) -> (-61.783, 49.2726) centre (-58.383, 49.2726) ccw projected
  line L9 (-58.383, 52.6726) -> (20.3726, 52.6726) projected
  arc A2 (23.7726, 49.2726) -> (20.3726, 52.6726) centre (20.3726, 49.2726) ccw projected
  line L10 (23.7726, 49.2726) -> (23.7726, -0.283) projected
  arc A3 (20.3726, -3.683) -> (23.7726, -0.283) centre (20.3726, -0.283) ccw projected
  line L11 (0.5726, -9.883) -> (0.5726, -7.283) projected
  line L12 (0.5726, -7.283) -> (6.3726, -7.283) projected
  line L13 (6.3726, -7.283) -> (6.3726, -9.883) projected
  line L14 (6.3726, -9.883) -> (23.7726, -9.883) projected
  line L15 (23.7726, -9.883) -> (23.7726, -11.683) projected
  line L16 (23.7726, -11.683) -> (-4.2274, -11.683) projected
  line L17 (-4.2274, -11.683) -> (-4.2274, -9.883) projected
  line L18 (-4.2274, -9.883) -> (0.5726, -9.883) projected
  line L19 (25.3726, -12.083) -> (25.3726, 49.2726) projected
  arc A4 (25.3726, 49.2726) -> (20.3726, 54.2726) centre (20.3726, 49.2726) ccw projected
  line L20 (20.3726, 54.2726) -> (-58.383, 54.2726) projected
  arc A5 (-58.383, 54.2726) -> (-63.383, 49.2726) centre (-58.383, 49.2726) ccw projected
  line L21 (-63.383, 49.2726) -> (-63.383, -0.283) projected
  arc A6 (-63.383, -0.283) -> (-58.383, -5.283) centre (-58.383, -0.283) ccw projected
  line L22 (-58.383, -5.283) -> (-16.2274, -5.283) projected
  line L23 (-51.8157, 29.3882) -> (-69.5161, 29.3882)
  line L24 (-69.5161, 29.3882) -> (-69.5161, 14.3356)
  line L25 (-69.5161, 14.3356) -> (-51.8157, 14.3356)
  line L26 (-51.8157, 14.3356) -> (-51.8157, 29.3882)
  line L27 (-12.6228, -5.283) -> (-8.8274, -5.283) projected
  arc A7 (-5.8274, -8.283) -> (-8.8274, -5.283) centre (-8.8274, -8.283) ccw projected
  line L28 (-5.8274, -10.7871) -> (-12.6228, -5.283) projected
  arc A8 (-14.3392, -5.9518) -> (-16.2274, -5.283) centre (-16.2274, -8.283) ccw projected
  line L29 (-14.3392, -5.9518) -> (-5.6198, -13.0143) projected
  arc A9 (-5.6198, -13.0143) -> (-3.7315, -13.683) centre (-3.7315, -10.683) ccw projected
  line L30 (-3.7315, -13.683) -> (23.7726, -13.683) projected
  arc A10 (23.7726, -13.683) -> (25.3726, -12.083) centre (23.7726, -12.083) ccw projected
  point P0 (-61.383, 0)
  point P1 (-61.783, 29.0882)
  point P2 (-61.783, 29.3882)
  point P3 (-63.383, 29.3882)
  point P4 (-63.383, 14.3356)
  point P5 (-61.783, 14.3356)
  point P6 (-61.783, 22.8624)
  dimension "d143" = 0.3
  dimension "d144" = 0.3
  constraints: 8 end point, 2 parallel, 1 horizontal, 1 perpendicular
  measures "d143" distance between parallel lines of L4 L23
  measures "d144" distance between parallel lines of L25 L0
extrude "Extrusion11" cut sketch "Skizze13" against normal blind 2.6 contours L8 L25 L21 L23 L4 L3 L2 | L2 L3 L4 L8
chamfer "Fase6" distance 1.2 angle 45 1 edges at (2, 21.8619, 1.4)
sketch "Skizze14" plane through (-61.383, 0, -1.2) normal (0, 0, -1) x (-1, 0, 0)
  line L0 (-61.783, 14.3356) -> (-63.383, 14.3356) projected
  line L1 (-63.383, 14.3356) -> (-63.383, -0.283) projected
  arc A0 (-63.383, -0.283) -> (-58.383, -5.283) centre (-58.383, -0.283) ccw projected
  line L2 (-58.383, -5.283) -> (-16.2274, -5.283) projected
  arc A1 (-14.3392, -5.9518) -> (-16.2274, -5.283) centre (-16.2274, -8.283) ccw projected
  line L3 (-14.3392, -5.9518) -> (-5.6198, -13.0143) projected
  arc A2 (-5.6198, -13.0143) -> (-3.7315, -13.683) centre (-3.7315, -10.683) ccw projected
  line L4 (-3.7315, -13.683) -> (23.7726, -13.683) projected
  arc A3 (23.7726, -13.683) -> (25.3726, -12.083) centre (23.7726, -12.083) ccw projected
  line L5 (25.3726, -12.083) -> (25.3726, 49.2726) projected
  arc A4 (25.3726, 49.2726) -> (20.3726, 54.2726) centre (20.3726, 49.2726) ccw projected
  line L6 (20.3726, 54.2726) -> (-58.383, 54.2726) projected
  arc A5 (-58.383, 54.2726) -> (-63.383, 49.2726) centre (-58.383, 49.2726) ccw projected
  line L7 (-63.383, 49.2726) -> (-63.383, 29.3882) projected
  line L8 (-63.383, 29.3882) -> (-61.783, 29.3882) projected
  line L9 (-61.783, 29.3882) -> (-61.783, 49.2726) projected
  arc A6 (-58.383, 52.6726) -> (-61.783, 49.2726) centre (-58.383, 49.2726) ccw projected
  line L10 (-58.383, 52.6726) -> (20.3726, 52.6726) projected
  arc A7 (23.7726, 49.2726) -> (20.3726, 52.6726) centre (20.3726, 49.2726) ccw projected
  line L11 (23.7726, 49.2726) -> (23.7726, -0.283) projected
  arc A8 (20.3726, -3.683) -> (23.7726, -0.283) centre (20.3726, -0.283) ccw projected
  line L12 (20.3726, -3.683) -> (-58.383, -3.683) projected
  arc A9 (-61.783, -0.283) -> (-58.383, -3.683) centre (-58.383, -0.283) ccw projected
  line L13 (-61.783, -0.283) -> (-61.783, 14.3356) projected
  line L14 (-12.6228, -5.283) -> (-8.8274, -5.283) projected
  arc A10 (-5.8274, -8.283) -> (-8.8274, -5.283) centre (-8.8274, -8.283) ccw projected
  line L15 (-5.8274, -8.283) -> (-5.8274, -10.7871) projected
  line L16 (-5.8274, -10.7871) -> (-12.6228, -5.283) projected
  line L17 (0.5726, -9.883) -> (0.5726, -7.283) projected
  line L18 (0.5726, -7.283) -> (6.3726, -7.283) projected
  line L19 (6.3726, -7.283) -> (6.3726, -9.883) projected
  line L20 (6.3726, -9.883) -> (23.7726, -9.883) projected
  line L21 (23.7726, -9.883) -> (23.7726, -11.683) projected
  line L22 (23.7726, -11.683) -> (-4.2274, -11.683) projected
  line L23 (-4.2274, -11.683) -> (-4.2274, -9.883) projected
  line L24 (-4.2274, -9.883) -> (0.5726, -9.883) projected
  line L25 (-5.8274, -10.7871) -> (-5.8274, -3.683)
  line L26 (20.3726, -3.683) -> (-58.383, -3.683) projected
  line L27 (-5.8274, -10.7871) -> (-12.6228, -5.283) projected
  line L28 (-12.6228, -5.283) -> (-13.3321, -4.7085)
  line L29 (-16.2274, -3.683) -> (-22.4657, -3.683)
  line L30 (-58.383, -3.683) -> (20.3726, -3.683) projected
  arc A11 (-13.3321, -4.7085) -> (-16.2274, -3.683) centre (-16.2274, -8.283) ccw
  point P0 (-61.383, 0)
  point P1 (-14.5981, -3.683)
  point P2 (-16.2274, -3.683)
  dimension "d150" = 3
  dimension "d151" = 4.6
  dimension "d152" = 1.6
  constraints: 6 end point, 5 point on line, 2 collinear, 2 point on circle, 2 tangent, 1 centre point, 1 perpendicular
  measures "d150" radius of A1
  measures "d151" radius of A11
  measures "d152" distance between parallel lines of L3 L16
extrude "Extrusion12" cut sketch "Skizze14" against normal up to surface (5 mm away) contours L12 L25 A10 L14 L28 A11 | L15 L16 L14 A10
fillet "Rundung4" radius 3 1 edges at (-55.5557, -3.683, 1.3)
chamfer "Fase7" distance 0.4 angle 45 8 edges at (-61.383, 51.35, 8.6) (-61.383, 2.35, 8.6) (-3.383, 2.35, 8.6) (-3.383, 51.35, 8.6) (-5, 40.9948, 8.6) (-5, 9.4948, 8.6) (-78.7557, 9.4948, 8.6) (-78.7557, 40.9948, 8.6)
equation "\"d1\" = d0"
equation "\"d2\" = d0"
equation "\"d3\" = d0"
equation "\"d4\" = d0"
equation "\"d5\" = d0"
equation "\"d6\" = d0"
equation "\"d7\" = d0"
equation "\"d14\" = d13"
equation "\"d17\" = d16"
equation "\"d21\" = d20"
equation "\"d22\" = d20"
equation "\"d23\" = d20"
equation "\"d25\" = d20"
equation "\"d40\" = d39"
equation "\"d41\" = d39"
equation "\"d42\" = d39"
equation "\"d43\" = d39"
equation "\"d44\" = d39"
equation "\"d45\" = d39"
equation "\"d46\" = d39"
equation "\"d47\" = d39"
equation "\"d48\" = d39"
equation "\"d49\" = d39"
equation "\"d55\" = d54"
equation "\"d56\" = d54"
equation "\"d57\" = d54"
equation "\"d58\" = d54"
equation "\"d59\" = d54"
equation "\"d60\" = d54"
equation "\"d61\" = d54"
equation "\"d62\" = d54"
equation "\"d63\" = d54"
equation "\"d64\" = d39"
equation "\"d65\" = d54"
equation "\"d66\" = d67"
equation "\"d69\" = d70"
